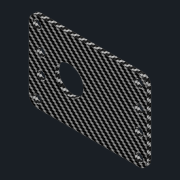
# Autodesk Inventor part: s_carbon_plate4
Saved by Autodesk Inventor 2022 (Build 260153000, 153)
## iProperties
Created: 2021-08-27
Part Number: s_carbon_plate4
Material: CFRP
Document SubType Name: Sheet Metal
Designer: Yuta Kage
Density: 1.43 g/cm^3
Sheet Metal Rule: Default_mm
Appearance: カーボンファイバー
Author: Yuta Kage
Autodesk Inventor part; units mm, degrees
ref_plane "YZ Plane" through (0, 0, 0) normal (1, 0, 0) x (0, 1, 0)
ref_plane "XZ Plane" through (0, 0, 0) normal (0, 1, 0) x (-1, 0, 0)
ref_plane "XY Plane" through (0, 0, 0) normal (0, 0, 1) x (1, 0, 0)
sketch "スケッチ1" plane through (0, 0, 0) normal (0, 0, 1) x (1, 0, 0)
  line L0 (-30, -20) -> (28.6, -20)
  line L1 (28.6, -20) -> (28.6, 20)
  line L2 (28.6, 20) -> (-30, 20)
  line L3 (-30, 20) -> (-30, -20)
  point P0 (0, 0)
  dimension "d1" = 40
  dimension "d28" = 30
  dimension "d29" = 28.6
  dimension "d32" = 20
  measures "d1" distance of L2.end L0.start
  measures "d28" distance from line of point (0, 0) L3
  measures "d29" distance from line of L1 point (0, 0)
  measures "d32" distance from line of point (0, 0) L2
extrude "プレート1" add sketch "スケッチ1" along normal blind 2
sketch "スケッチ2" plane through (0, 0, 2) normal (0, 0, 1) x (1, 0, 0)
  line L0 (-24, -5) -> (24.6, -5)
  line L1 (24.6, -5) -> (24.6, 5)
  line L2 (24.6, 5) -> (-24, 5)
  line L3 (-24, 5) -> (-24, -5)
  line L4 (-24, -5) -> (24.6, 5) construction
  line L5 (24.6, -5) -> (-24, 5) construction
  line L6 (28.6, -20) -> (-30, -20) projected
  line L7 (-30, -20) -> (-30, 20) projected
  line L8 (28.6, -20) -> (-30, -20) projected
  line L9 (28.6, 20) -> (28.6, -20) projected
  line L10 (-30, 20) -> (28.6, 20) projected
  circle A0 centre (-10, 0) radius 7
  point P0 (0.3, 0)
  point P1 (0.3, 0)
  point P2 (0.3, 0)
  point P3 (0, 0)
  dimension "d3" = 48.6
  dimension "d5" = 10
  dimension "d8" = 20
  dimension "d16" = 14
  dimension "d30" = 20
  dimension "d31" = 14
  constraints: 12 end point, 4 midpoint, 2 parallel, 1 centre point, 1 coincident, 1 horizontal, 1 horizontal alignment, 1 perpendicular
  measures "d3" distance of L1.end L2.end
  measures "d5" distance of L0.end L1.end
  measures "d8" distance from line of L6 point (0.3, 0)
  measures "d16" diameter of A0
  measures "d30" distance from line of L7 A0.centre
  measures "d31" distance from line of L3 A0.centre
hole "穴1" at (24.6, 5, 2) at (24.6, -5, 2) at (-24, 5, 2) at (-24, -5, 2) direction (0, 0, -1) diameter 4.3 end through all clearance for "Socket Head Cap Screw" size "M4" standard "Ansi Metric M Profile"
extrude "押し出し1" cut sketch "スケッチ2" against normal blind 10 contours A0 L2 L0 | L0 A0 | A0 L2
sketch "スケッチ3" plane through (0, 0, 2) normal (0, 0, 1) x (1, 0, 0)
  line L0 (-30, 20) -> (28.6, 20) projected
  line L1 (-30, -20) -> (-30, 20) projected
  line L2 (28.6, -20) -> (-30, -20) projected
  line L3 (28.6, 20) -> (28.6, -20) projected
  line L4 (24.6, 16) -> (-26, 16)
  line L5 (-26, 16) -> (-26, -16)
  line L6 (-26, -16) -> (24.6, -16)
  line L7 (24.6, -16) -> (24.6, 16)
  point P0 (0, 0)
  dimension "d19" = 4
  constraints: 8 end point, 3 other
  measures "d19" distance between parallel lines of L0 L4
hole "穴2" at (-26, 16, 2) at (-26, -16, 2) at (24.6, 16, 2) at (24.6, -16, 2) direction (0, 0, -1) diameter 4.3 end through all clearance for "Socket Head Cap Screw" size "M4" standard "Ansi Metric M Profile"
fillet "コーナーR1" radius 4 4 edges at (28.6, 20, 1) (-30, 20, 1) (-30, -20, 1) (28.6, -20, 1)
equation "\"d14\" = Thickness"
equation "\"d2\" = Thickness"
equation "\"BendRadius\" = Thickness"
equation "\"BendReliefWidth\" = Thickness"
equation "\"BendReliefDepth\" = 0.5 * Thickness"
equation "\"CornerReliefSize\" = 4 * Thickness"
equation "\"MinimumRemnant\" = 2 * Thickness"
equation "\"TransitionRadius\" = BendRadius"
equation "\"JacobiRadiusSize\" = BendRadius"
equation "\"GapSize\" = Thickness"
equation "\"Thickness\" = 2"
